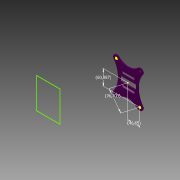
# Autodesk Inventor part: BAWAH4
Saved by Autodesk Inventor 2015 (Build 190159000, 159)
## iProperties
Created: 2015-01-14
Part Number: BAWAH4
Material: Generic
Document SubType Name: Modeling
Designer: Rafi Kurnia Putra
Density: 1 g/cm^3
Appearance: Smooth - Purple
Author: Rafi Kurnia Putra
Autodesk Inventor part; units mm, degrees
ref_plane "YZ Plane" through (0, 0, 0) normal (1, 0, 0) x (0, 1, 0)
ref_plane "XZ Plane" through (0, 0, 0) normal (0, 1, 0) x (-1, 0, 0)
ref_plane "XY Plane" through (0, 0, 0) normal (0, 0, 1) x (1, 0, 0)
sketch "Sketch1" plane through (0, 0, 0) normal (0, 1, 0) x (-1, 0, 0)
  arc A0 (39.6019, 0) -> (55.3297, -52.2069) centre (134.1138, 0) ccw
  circle A1 centre (28.625, -37.55) radius 1.75
  circle A2 centre (25.375, -42.175) radius 1.75
  circle A3 centre (46.65, -60.8866) radius 4.25
  arc A4 (37.9702, -69.5664) -> (55.3297, -52.2069) centre (46.65, -60.8866) ccw
  arc A5 (37.9702, -69.5664) -> (0, -53.8386) centre (0, -107.5366) ccw
  line L0 (28.315, -9.4519) -> (0.0544, -9.4519)
  arc A6 (28.315, -9.4519) -> (28.625, -9.4382) centre (28.315, -5.9519) ccw
  arc A7 (28.315, -9.4519) -> (31.815, -5.9519) centre (28.315, -5.9519) ccw
  line L1 (31.815, 0) -> (31.815, -5.9519)
  circle A8 centre (46.65, -60.8866) radius 4.25
  circle A9 centre (25.375, -42.175) radius 1.75
  circle A10 centre (28.625, -37.55) radius 1.75
  arc A11 (39.6019, 0) -> (55.3297, -52.2069) centre (134.1138, 0) ccw
  arc A12 (37.9702, -69.5664) -> (0, -53.8386) centre (0, -107.5366) ccw
  line L2 (39.6019, 0) -> (0, 0) construction
  line L3 (0, -18.3592) -> (21.875, -18.3592)
  line L4 (25.375, -21.8592) -> (25.375, -24.8427)
  line L5 (21.875, -28.3427) -> (0, -28.3427)
  arc A13 (25.375, -21.8592) -> (21.875, -18.3592) centre (21.875, -21.8592) ccw
  arc A14 (21.875, -28.3427) -> (25.375, -24.8427) centre (21.875, -24.8427) ccw
  arc A15 (0, -42.175) -> (0, -38.675) centre (0, -40.425) ccw
  line L6 (0, -53.8386) -> (0, -42.175) construction
  line L7 (31.815, 0) -> (31.815, 5.9519)
  arc A16 (31.815, 5.9519) -> (28.315, 9.4519) centre (28.315, 5.9519) ccw
  arc A17 (28.625, 9.4382) -> (28.315, 9.4519) centre (28.315, 5.9519) ccw
  line L8 (28.315, 9.4519) -> (0.0544, 9.4519)
  arc A18 (55.3297, 52.2069) -> (39.6019, 0) centre (134.1138, 0) ccw
  circle A19 centre (28.625, 37.55) radius 1.75
  circle A20 centre (25.375, 42.175) radius 1.75
  arc A21 (0, 53.8386) -> (37.9702, 69.5664) centre (0, 107.5366) ccw
  circle A22 centre (46.65, 60.8866) radius 4.25
  arc A23 (55.3297, 52.2069) -> (37.9702, 69.5664) centre (46.65, 60.8866) ccw
  circle A24 centre (46.65, 60.8866) radius 4.25
  circle A25 centre (25.375, 42.175) radius 1.75
  circle A26 centre (28.625, 37.55) radius 1.75
  arc A27 (55.3297, 52.2069) -> (39.6019, 0) centre (134.1138, 0) ccw
  arc A28 (0, 53.8386) -> (37.9702, 69.5664) centre (0, 107.5366) ccw
  line L9 (0, 18.3592) -> (21.875, 18.3592)
  line L10 (25.375, 21.8592) -> (25.375, 24.8427)
  line L11 (21.875, 28.3427) -> (0, 28.3427)
  arc A29 (21.875, 18.3592) -> (25.375, 21.8592) centre (21.875, 21.8592) ccw
  arc A30 (25.375, 24.8427) -> (21.875, 28.3427) centre (21.875, 24.8427) ccw
  arc A31 (0, 38.675) -> (0, 42.175) centre (0, 40.425) ccw
  line L12 (0, 53.8386) -> (0, 42.175) construction
  line L13 (0, 38.675) -> (0, 0) construction
  line L14 (-31.815, 0) -> (-31.815, -5.9519)
  arc A32 (-31.815, -5.9519) -> (-28.315, -9.4519) centre (-28.315, -5.9519) ccw
  arc A33 (-28.625, -9.4382) -> (-28.315, -9.4519) centre (-28.315, -5.9519) ccw
  line L15 (-28.315, -9.4519) -> (-0.0544, -9.4519)
  arc A34 (-55.3297, -52.2069) -> (-39.6019, 0) centre (-134.1138, 0) ccw
  circle A35 centre (-28.625, -37.55) radius 1.75
  circle A36 centre (-25.375, -42.175) radius 1.75
  arc A37 (0, -53.8386) -> (-37.9702, -69.5664) centre (0, -107.5366) ccw
  circle A38 centre (-46.65, -60.8866) radius 4.25
  arc A39 (-55.3297, -52.2069) -> (-37.9702, -69.5664) centre (-46.65, -60.8866) ccw
  circle A40 centre (-46.65, -60.8866) radius 4.25
  circle A41 centre (-25.375, -42.175) radius 1.75
  circle A42 centre (-28.625, -37.55) radius 1.75
  arc A43 (-55.3297, -52.2069) -> (-39.6019, 0) centre (-134.1138, 0) ccw
  arc A44 (0, -53.8386) -> (-37.9702, -69.5664) centre (0, -107.5366) ccw
  line L16 (0, -18.3592) -> (-21.875, -18.3592)
  line L17 (-25.375, -21.8592) -> (-25.375, -24.8427)
  line L18 (-21.875, -28.3427) -> (0, -28.3427)
  arc A45 (-21.875, -18.3592) -> (-25.375, -21.8592) centre (-21.875, -21.8592) ccw
  arc A46 (-25.375, -24.8427) -> (-21.875, -28.3427) centre (-21.875, -24.8427) ccw
  arc A47 (0, -38.675) -> (0, -42.175) centre (0, -40.425) ccw
  line L19 (0, 18.3592) -> (-21.875, 18.3592)
  arc A48 (-25.375, 21.8592) -> (-21.875, 18.3592) centre (-21.875, 21.8592) ccw
  line L20 (-28.315, 9.4382) -> (-0.0544, 9.445)
  arc A49 (-28.315, 9.4382) -> (-31.815, 5.9519) centre (-28.315, 5.9382) ccw
  line L21 (-31.815, 0) -> (-31.815, 5.9519)
  arc A50 (-28.315, 9.4382) -> (-28.6259, 9.4244) centre (-28.315, 5.9382) ccw
  arc A51 (-37.9702, 69.5664) -> (0, 53.8386) centre (0, 107.5366) ccw
  arc A52 (-37.9702, 69.5664) -> (0, 53.8386) centre (0, 107.5366) ccw
  circle A53 centre (-46.65, 60.8866) radius 4.25
  circle A54 centre (-46.65, 60.8866) radius 4.25
  arc A55 (-37.9702, 69.5664) -> (-55.3297, 52.2069) centre (-46.65, 60.8866) ccw
  arc A56 (-21.875, 28.3427) -> (-25.375, 24.8427) centre (-21.875, 24.8427) ccw
  circle A57 centre (-28.625, 37.55) radius 1.75
  circle A58 centre (-25.375, 42.175) radius 1.75
  circle A59 centre (-25.375, 42.175) radius 1.75
  line L22 (-21.875, 28.3427) -> (0, 28.3427)
  arc A60 (0, 42.175) -> (0, 38.675) centre (0, 40.425) ccw
  arc A61 (-39.6019, 0) -> (-55.3297, 52.2069) centre (-134.1138, 0) ccw
  circle A62 centre (-28.625, 37.55) radius 1.75
  line L23 (-25.375, 21.8592) -> (-25.375, 24.8427)
  arc A63 (-39.6019, 0) -> (-55.3297, 52.2069) centre (-134.1138, 0) ccw
  circle A64 centre (-25.5, 34.24) radius 1.75
  circle A65 centre (-25.5, -34.24) radius 1.75
  circle A66 centre (25.5, 34.24) radius 1.75
  circle A67 centre (25.5, -34.24) radius 1.75
  arc A68 (-37.9702, 69.5664) -> (-55.3297, 52.2069) centre (-46.65, 60.8866) ccw
  arc A69 (-55.3297, -52.2069) -> (-37.9702, -69.5664) centre (-46.65, -60.8866) ccw
  arc A70 (55.3297, 52.2069) -> (37.9702, 69.5664) centre (46.65, 60.8866) ccw
  arc A71 (37.9702, -69.5664) -> (55.3297, -52.2069) centre (46.65, -60.8866) ccw
  arc A72 (-37.9702, 69.5664) -> (37.9702, 69.5664) centre (0, 107.5366) ccw
  arc A73 (37.9702, -69.5664) -> (-37.9702, -69.5664) centre (0, -107.5366) ccw
  arc A74 (-55.3297, -52.2069) -> (-55.3297, 52.2069) centre (-134.1138, 0) ccw
  arc A75 (55.3297, 52.2069) -> (55.3297, -52.2069) centre (134.1138, 0) ccw
  line L24 (-21.875, 28.3427) -> (21.875, 28.3427)
  line L25 (21.875, 18.3592) -> (-21.875, 18.3592)
  line L26 (-25.375, 24.8427) -> (-25.375, 21.8592)
  line L27 (25.375, 24.8427) -> (25.375, 21.8592)
  line L28 (-28.315, 9.4382) -> (28.625, 9.4382)
  line L29 (28.625, -9.4382) -> (-28.625, -9.4382)
  line L30 (-31.815, 5.9519) -> (-31.815, -5.9519)
  line L31 (31.815, 5.9519) -> (31.815, -5.9519)
  line L32 (-21.875, -18.3592) -> (21.875, -18.3592)
  line L33 (21.875, -28.3427) -> (-21.875, -28.3427)
  line L34 (-25.375, -21.8592) -> (-25.375, -24.8427)
  line L35 (25.375, -21.8592) -> (25.375, -24.8427)
  arc A76 (-21.875, 28.3427) -> (-25.375, 24.8427) centre (-21.875, 24.8427) ccw
  arc A77 (-25.375, 21.8592) -> (-21.875, 18.3592) centre (-21.875, 21.8592) ccw
  arc A78 (25.375, 24.8427) -> (21.875, 28.3427) centre (21.875, 24.8427) ccw
  arc A79 (21.875, 18.3592) -> (25.375, 21.8592) centre (21.875, 21.8592) ccw
  circle A80 centre (0, 40.425) radius 1.75
  circle A81 centre (0, -40.425) radius 1.75
  point P0 (55.3297, 52.2069)
  point P1 (25.25, -18.3592)
  point P2 (4.2075, -54.5249)
  point P3 (-37.9702, -69.5664)
  point P4 (25.25, 18.3592)
  point P5 (4.2075, 54.5249)
  point P6 (-25.25, -18.3592)
  point P7 (-4.2075, -54.5249)
  point P8 (-25.25, 18.3592)
  point P9 (-4.2075, 54.5249)
  dimension "d93" = 3.5
  dimension "d94" = 37.55
  dimension "d95" = 4.625
  dimension "d96" = 3.5
  dimension "d97" = 3.5
  dimension "d98" = 8.5
  dimension "d100" = 3.5
  dimension "d105" = 3.5
  dimension "d106" = 3.5
  dimension "d107" = 3.5
  dimension "d108" = 3.5
  constraints: 126 point on circle, 82 centre point, 72 end point, 32 symmetric about line, 18 coincident, 12 equal radius, 8 tangent, 5 collinear, 5 parallel, 3 horizontal, 3 perpendicular, 1 point on line, 1 vertical, 16 other
  measures "d93" radius of A13
  measures "d94" distance from line of A1.centre L2
  measures "d95" vertical distance of A2.centre A1.centre
  measures "d96" diameter of A2
  measures "d97" diameter of A1
  measures "d98" diameter of A3
  measures "d100" diameter of A15
  measures "d105" diameter of A64
  measures "d106" diameter of A65
  measures "d107" diameter of A66
  measures "d108" diameter of A67
extrude "Extrusion7" add sketch "Sketch1" along normal blind 3.5
sketch "Sketch8" plane through (0, 0, 0) normal (0, -1, 0) x (1, 0, 0)
  circle A0 centre (35.7085, -13.8987) radius 1.75
  circle A1 centre (-35.7085, -13.8987) radius 1.75
  circle A2 centre (35.7085, 13.8987) radius 1.75
  circle A3 centre (-35.7085, 13.8987) radius 1.75
  circle A4 centre (46.65, -60.8866) radius 4.25 projected
  dimension "d120" = 46.9879
  dimension "d121" = 10.9415
  constraints: 4 centre point
  measures "d120" vertical distance of A0.centre A4.centre
  measures "d121" horizontal distance of A0.centre A4.centre
extrude "Extrusion8" cut sketch "Sketch8" against normal through all contours A0 | A1 | A2 | A3
sketch "Sketch11" plane through (0, 0, 0) normal (0, -1, 0) x (1, 0, 0)
  circle A0 centre (46.65, -60.8866) radius 4.25 projected
  circle A1 centre (-46.65, 60.8866) radius 4.25 projected
  line L0 (-363.8211, -156.3161) -> (-270.5212, -156.3161)
  line L1 (-270.5212, -156.3161) -> (-270.5212, -277.4814)
  line L2 (-270.5212, -277.4814) -> (-363.8211, -277.4814)
  line L3 (-363.8211, -277.4814) -> (-363.8211, -156.3161)
  point P0 (0, 0)
  dimension "d122" = 76.7033
  dimension "d123" = 60.8866
  dimension "d124" = 46.65
  constraints: 8 end point, 2 parallel, 1 horizontal, 1 perpendicular
  measures "d122" distance of point (0, 0) A0.centre
  measures "d123" vertical distance of point (0, 0) A0.centre
  measures "d124" horizontal distance of A0.centre point (0, 0)
body "Solid4"
